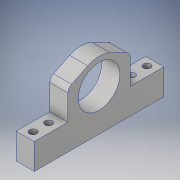
# Autodesk Inventor part: Bearing Block
Saved by Autodesk Inventor 2019.4 (Build 234330000, 330)
## iProperties
Created: 2020-01-06
Part Number: Bearing Block
Material: Aluminum 6061
Document SubType Name: Modeling
Designer: admin
Density: 2.7 g/cm^3
Appearance: Aluminum - Flat
Author: admin
Autodesk Inventor part; units mm, degrees
ref_plane "YZ Plane" through (0, 0, 0) normal (1, 0, 0) x (0, 1, 0)
ref_plane "XZ Plane" through (0, 0, 0) normal (0, 1, 0) x (-1, 0, 0)
ref_plane "XY Plane" through (0, 0, 0) normal (0, 0, 1) x (1, 0, 0)
sketch "Sketch1" plane through (0, 0, 0) normal (1, 0, 0) x (0, 1, 0)
  circle A0 centre (0, 0) radius 16
  arc A1 (17.9987, 8.7204) -> (17.9987, -8.7204) centre (0, 0) ccw construction
  line L0 (17.9987, 8.7204) -> (-2.0013, 50)
  line L1 (-2.0013, 50) -> (-32, 50)
  line L2 (-32, 50) -> (-32, -50)
  line L3 (-32, -50) -> (-2.0013, -50)
  line L4 (-2.0013, -50) -> (17.9987, -8.7204)
  arc A2 (17.9987, -8.7204) -> (17.9987, 8.7204) centre (0, 0) ccw
  dimension "d0" = 32
  dimension "d1" = 40
  dimension "d2" = 100
  dimension "d5" = 32
  dimension "d6" = 20
  constraints: 10 end point, 4 point on circle, 3 centre point, 2 coincident, 2 equal length, 2 perpendicular, 2 tangent, 1 horizontal
  measures "d0" diameter of A0
  measures "d1" diameter of A1
  measures "d2" distance of L1.end L2.end
  measures "d5" distance from line of L2 point (0, 0)
  measures "d6" horizontal distance of L0.start L0.end
extrude "Extrusion1" add sketch "Sketch1" along normal blind 14
sketch "Sketch2" plane through (0, -32, -50) normal (0, -1, 0) x (1, 0, 0)
  circle A0 centre (7, 94) radius 2.75
  circle A1 centre (7, 6) radius 2.75
  circle A2 centre (7, 18) radius 2.75
  circle A3 centre (7, 82) radius 2.75
  line L0 (0, 100) -> (0, 0) projected
  line L1 (0, 100) -> (14, 100) projected
  line L2 (0, 0) -> (14, 0) projected
  point P0 (0, 50)
  dimension "d9" = 5.5
  dimension "d10" = 5.5
  dimension "d11" = 5.5
  dimension "d12" = 5.5
  dimension "d13" = 7
  dimension "d14" = 7
  dimension "d15" = 7
  dimension "d16" = 7
  dimension "d17" = 12
  dimension "d18" = 6
  dimension "d19" = 6
  dimension "d20" = 12
  constraints: 4 centre point
  measures "d9" diameter of A0
  measures "d10" diameter of A1
  measures "d11" diameter of A2
  measures "d12" diameter of A3
  measures "d13" distance from line of L0 A0.centre
  measures "d14" distance from line of L0 A3.centre
  measures "d15" distance from line of L0 A1.centre
  measures "d16" distance from line of L0 A2.centre
  measures "d17" distance of A3.centre A0.centre
  measures "d18" distance from line of L1 A0.centre
  measures "d19" distance from line of L2 A1.centre
  measures "d20" distance of A1.centre A2.centre
extrude "Extrusion2" cut sketch "Sketch2" against normal through all
ref_plane "Work Plane1" through (0, -12, -50) normal (0, -1, 0) x (1, 0, 0)
sketch "Sketch3" plane through (0, -12, -50) normal (0, -1, 0) x (1, 0, 0)
  circle A0 centre (7, 94) radius 2.75 projected
  circle A1 centre (7, 82) radius 2.75 projected
  line L0 (0, 58.7204) -> (0, 100) projected
  line L1 (0, 100) -> (14, 100) projected
  line L2 (14, 58.7204) -> (14, 100) projected
  line L3 (0, 58.7204) -> (14, 58.7204) projected
  circle A2 centre (7, 18) radius 2.75 projected
  circle A3 centre (7, 6) radius 2.75 projected
  line L4 (0, 0) -> (0, 41.2796) projected
  line L5 (0, 41.2796) -> (14, 41.2796) projected
  line L6 (14, 0) -> (14, 41.2796) projected
  line L7 (0, 0) -> (14, 0) projected
  line L8 (14, 100) -> (14, 0) projected
  line L9 (0, 58.7204) -> (0, 100) projected
  line L10 (0, 74) -> (14, 74)
  line L11 (0, 26) -> (14, 26)
  point P0 (0, 50)
  dimension "d27" = 8
  dimension "d28" = 8
  constraints: 4 end point, 4 point on line, 2 perpendicular
  measures "d27" distance from line of A2.centre L11
  measures "d28" distance from line of A1.centre L10
extrude "Extrusion3" cut sketch "Sketch3" against normal through all contours L0 L1 L2 L10 | L4 L11 L6 L7
fillet "Fillet2" radius 5 2 edges at (7, 10.5958, 24) (7, 10.5958, -24)
body "Solid1"
